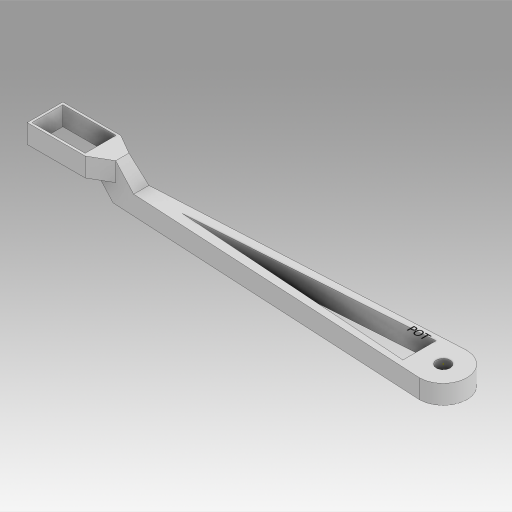
# Autodesk Inventor part: pointrer
Saved by Autodesk Inventor 2024.3 (Build 283343000, 343)
## iProperties
Created: 2024-07-21
Part Number: pointrer
Material: Ogólny
Document SubType Name: Modeling
Designer: User
Density: 1 g/cm^3
Appearance: Domyślna
Author: User
Autodesk Inventor part; units mm, degrees
ref_plane "YZ Plane" through (0, 0, 0) normal (1, 0, 0) x (0, 1, 0)
ref_plane "XZ Plane" through (0, 0, 0) normal (0, 1, 0) x (-1, 0, 0)
sketch "Szkic1" plane through (-150, 0, 2) normal (0, -1, 0) x (1, 0, 0)
  circle A0 centre (150, -2) radius 2.4
  line L0 (150, -2) -> (150, 8)
  line L1 (150, -2) -> (150, -12)
  arc A1 (150, -12) -> (150, 8) centre (150, -2) ccw
  line L2 (150, -2) -> (0, -2)
  line L3 (150, -2) -> (300, -2) construction
  line L4 (0, -2) -> (0, 0)
  line L5 (0, -2) -> (0, -4)
  line L6 (0, -4) -> (150, -12)
  line L7 (0, 0) -> (150, 8)
  dimension "d0" = 4.8
  dimension "d1" = 10
  dimension "d2" = 10
  dimension "d3" = 150
  dimension "d4" = 180
  dimension "d5" = 2
  dimension "d6" = 2
  constraints: 16 end point, 4 vertical, 2 centre point, 2 horizontal, 2 point on circle, 1 coincident, 1 collinear
  measures "d0" diameter of A0
  measures "d1" distance of L0.start L0.end
  measures "d2" distance of L0.start L1.end
  measures "d3" distance of L2.start L2.end
  measures "d4" angle of L2 L3
  measures "d5" distance of L2.end L4.end
  measures "d6" distance of L2.end L5.end
extrude "Wyciągnięcie proste1" add sketch "Szkic1" against normal blind 8 contours A0 L0 A1 L1 | A0 L2 L4 L7 L0 | L1 L6 L5 L2 A0
sketch "Szkic2" plane through (-150, 8, 2) normal (0, 1, 0) x (1, 0, 0)
  circle A0 centre (150, 2) radius 2.4
  circle A1 centre (150, 2) radius 2.95
  dimension "d9" = 5.9
  constraints: 2 centre point, 2 coincident
  measures "d9" diameter of A1
extrude "Wyciągnięcie proste2" cut sketch "Szkic2" against normal blind 4
ref_plane "Płaszczyzna konstrukcyjna1" through (-150, 3.5, 2) normal (0, -1, 0) x (1, 0, 0)
sketch "Szkic4" plane through (-150, 3.5, 2) normal (0, -1, 0) x (1, 0, 0)
  circle A0 centre (150, -2) radius 1.5
  circle A1 centre (150, -2) radius 2.4
  dimension "d13" = 3
  constraints: 2 centre point, 2 coincident
  measures "d13" diameter of A0
extrude "Wyciągnięcie proste3" add sketch "Szkic4" along normal blind 1
sketch "Szkic5" plane through (-150, 8, 2) normal (0, 1, 0) x (1, 0, 0)
  line L0 (129.6292, 9.8056) -> (142.004, 9.8056) construction
  line L1 (142.004, 9.8056) -> (142.004, -5.0441) construction
  line L2 (142.004, -5.0441) -> (129.6292, -5.0441) construction
  line L3 (129.6292, -5.0441) -> (129.6292, 9.8056) construction
  point P0 (150, 2)
  constraints: 2 other
sketch "Szkic6" plane through (-150, 8, 2) normal (0, 1, 0) x (1, 0, 0)
  circle A0 centre (150, 2) radius 1.5 projected
  line L0 (150, 2) -> (0, 2)
  line L1 (150, 2) -> (300, 2) construction
  line L2 (0, 2) -> (5.6, 2)
  line L3 (5.6, 2) -> (-16.8, 2)
  line L4 (5.6, 2) -> (-16.8, 2)
  line L5 (-16.8, 2) -> (-16.8, -4.5)
  line L6 (-16.8, -4.5) -> (5.6, -4.5)
  line L7 (5.6, -4.5) -> (5.6, 2)
  line L8 (5.6, 2) -> (-16.8, 2)
  line L9 (-16.8, 2) -> (-16.8, 8.5)
  line L10 (-16.8, 8.5) -> (5.6, 8.5)
  line L11 (5.6, 8.5) -> (5.6, 2)
  line L12 (5.6, 8.5) -> (5.6, 9.5)
  line L13 (5.6, 9.5) -> (6.6, 9.5)
  line L14 (-16.8, -4.5) -> (-16.8, -5.5)
  line L15 (-16.8, -5.5) -> (-17.8, -5.5)
  line L16 (-17.8, -5.5) -> (6.6, -5.5)
  line L17 (6.6, -5.5) -> (6.6, 9.5)
  line L18 (6.6, 9.5) -> (-17.8, 9.5)
  line L19 (-17.8, 9.5) -> (-17.8, -5.5)
  line L20 (6.6, -5.5) -> (14.7626, -0.7873)
  line L21 (150, -8) -> (0, 0) projected
  line L22 (6.6, -5.5) -> (16.0253, -5.5) construction
  line L23 (6.6, 9.5) -> (14.7626, 4.7873)
  line L24 (14.7626, -0.7873) -> (14.7626, 4.7873)
  point P0 (5.6, 9.5)
  dimension "d16" = 150
  dimension "d17" = 180
  dimension "d18" = 5.6
  dimension "d19" = 22.4
  dimension "d20" = 6.5
  dimension "d21" = 6.5
  dimension "d22" = 1
  dimension "d23" = 1
  dimension "d24" = 1
  dimension "d25" = 1
  dimension "d26" = 30
  constraints: 48 end point, 7 horizontal, 6 parallel, 5 perpendicular, 3 point on line, 3 vertical, 2 equal length, 1 symmetric about line
  measures "d16" distance of L0.start L0.end
  measures "d17" angle of L0 L1
  measures "d18" distance of L0.end L2.end
  measures "d19" distance of L2.end L3.end
  measures "d20" distance of L5.end L4.end
  measures "d21" distance of L8.end L9.end
  measures "d22" distance of L10.end L12.end
  measures "d23" distance of L12.end L13.end
  measures "d24" distance of L5.end L14.end
  measures "d25" distance of L14.end L15.end
  measures "d26" angle of L22 L20
extrude "Wyciągnięcie proste4" add sketch "Szkic6" along normal blind 8 contours L11 L12 L13 L17 L0 | L0 L17 L21 L7 | L17 L23 L24 L0 | L0 L24 L21 L17 | L21 L17 L16 L14 L6 L7 | L10 L9 L5 L14 L15 L19 L18 L12 | L21 L20 L17
sketch "Szkic7" plane through (-150, 8, 2) normal (0, 1, 0) x (1, 0, 0)
  circle A0 centre (150, 2) radius 1.5 projected
  line L0 (150, 2) -> (140, 2)
  line L1 (140, 2) -> (140, -5)
  line L2 (140, 2) -> (140, 9)
  line L3 (140, 2) -> (40, 2)
  line L4 (40, 2) -> (140, 9)
  line L5 (40, 2) -> (140, -5)
  line L6 (5.6, -0.2987) -> (5.6, 4.2987) projected
  line L7 (5.6, 4.2987) -> (5.6, -0.2987)
  line L8 (0, 0) -> (5.6, -0.2987) projected
  line L9 (5.6, -0.2987) -> (0, 0)
  line L10 (0, 0) -> (0, 4.0412)
  line L11 (0, 4.0412) -> (5.6, 4.2987)
  dimension "d29" = 10
  dimension "d30" = 7
  dimension "d31" = 7
  dimension "d32" = 100
  constraints: 20 end point, 2 collinear, 2 perpendicular, 1 horizontal, 1 parallel, 1 vertical
  measures "d29" distance of L0.start L0.end
  measures "d30" distance of L0.end L1.end
  measures "d31" distance of L0.end L2.end
  measures "d32" distance of L0.end L3.end
extrude "Wyciągnięcie proste5" cut sketch "Szkic7" against normal through all contours L3 L4 L2 | L1 L5 L3 | L8 L10 L11 L6
chamfer "Faza1" distance 8 angle 45 1 edges at (-135.2374, 8, 0)
chamfer "Faza2" distance 8 angle 45 1 edges at (-144.4, 0, 0)
sketch "Szkic8" plane through (-150, 0, 2) normal (0, -1, 0) x (1, 0, 0)
  circle A0 centre (150, -2) radius 2.4 projected
  line L0 (150, -2) -> (0, -2)
  circle A1 centre (0, -2) radius 2
  dimension "d41" = 150
  dimension "d42" = 4
  constraints: 2 end point, 1 centre point, 1 coincident, 1 horizontal
  measures "d41" distance of L0.start L0.end
  measures "d42" diameter of A1
sketch "Szkic9" plane through (-150, 8, 2) normal (0, -1, 0) x (1, 0, 0)
  point P0 (150, -2)
sketch "Szkic10" plane through (-150, 0, 2) normal (0, -1, 0) x (1, 0, 0)
  circle A0 centre (150, -2) radius 2.85
  dimension "d43" = 5.7
  constraints: 1 centre point, 1 coincident
  measures "d43" diameter of A0
extrude "Wyciągnięcie proste6" cut sketch "Szkic10" against normal blind 2.5
